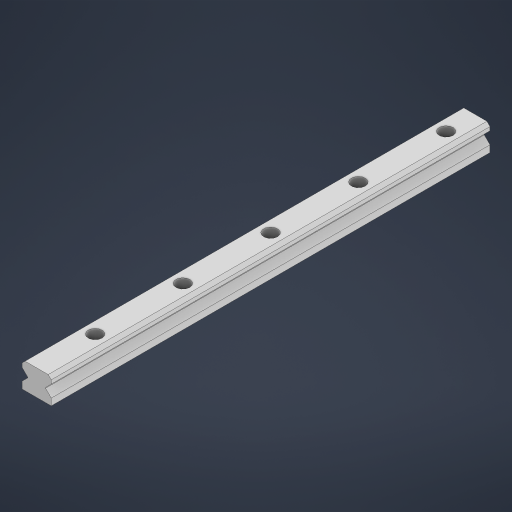
# Autodesk Inventor part: HGR20 500mm
Saved by Autodesk Inventor 2024.2 (Build 282272000, 272)
## iProperties
Created: 2024-10-04
Part Number: HGR20 500mm
Material: Generic
Document SubType Name: Modeling
Designer: jerem
Density: 1 g/cm^3
Appearance: Default
Author: jerem
Autodesk Inventor part; units mm, degrees
ref_plane "YZ Plane" through (0, 0, 0) normal (1, 0, 0) x (0, 1, 0)
ref_plane "XZ Plane" through (0, 0, 0) normal (0, 1, 0) x (-1, 0, 0)
ref_plane "XY Plane" through (0, 0, 0) normal (0, 0, 1) x (1, 0, 0)
sketch "Sketch1" plane through (0, 0, 0) normal (0, 0, 1) x (1, 0, 0)
  line L0 (0, 0) -> (0, 17.5) construction
  line L1 (0, 0) -> (-10, 0)
  line L2 (0, 0) -> (10, 0)
  line L3 (-10, 0) -> (-10, 4.6)
  line L4 (-10, 4.6) -> (-6.1, 8.5)
  line L5 (-6.1, 8.5) -> (-6.1, 9)
  line L6 (-6.1, 9) -> (-10, 12.9)
  line L7 (-10, 12.9) -> (-10, 15.4)
  line L8 (-10, 15.4) -> (-7.9, 17.5)
  line L9 (-7.9, 17.5) -> (0, 17.5)
  line L10 (10, 0) -> (10, 4.6)
  line L11 (10, 4.6) -> (6.1, 8.5)
  line L12 (6.1, 8.5) -> (6.1, 9)
  line L13 (6.1, 9) -> (10, 12.9)
  line L14 (10, 12.9) -> (10, 15.4)
  line L15 (10, 15.4) -> (7.9, 17.5)
  line L16 (7.9, 17.5) -> (0, 17.5)
  dimension "d0" = 17.5
  dimension "d1" = 20
  dimension "d2" = 4.6
  dimension "d3" = 8.5
  dimension "d8" = 135
  dimension "d9" = 0.5
  dimension "d10" = 135
  dimension "d11" = 2.5
  constraints: 34 end point, 6 symmetric about line, 4 point on line, 2 horizontal, 2 parallel, 2 vertical, 1 collinear, 1 perpendicular
  measures "d0" distance of L0.start L0.end
  measures "d1" distance of L2.end L1.end
  measures "d2" distance of L1.end L3.end
  measures "d3" distance from line of L5.end L9
  measures "d8" angle of L9 L8
  measures "d9" distance of L4.end L5.end
  measures "d10" angle of L5 L6
  measures "d11" distance of L6.end L7.end
extrude "Extrusion1" add sketch "Sketch1" along normal blind 300
sketch "Sketch2" plane through (0, 0, 0) normal (0, 1, 0) x (-1, 0, 0)
  line L0 (0, 0) -> (0, 20) construction
  line L1 (0, 20) -> (0, 80) construction
  circle A0 centre (0, 20) radius 4.75
  circle A1 centre (0, 20) radius 3
  dimension "d14" = 20
  dimension "d15" = 60
  dimension "d16" = 9.5
  dimension "d17" = 6
  constraints: 4 end point, 2 centre point, 2 coincident, 1 point on line, 1 vertical
  measures "d14" distance of L0.start L0.end
  measures "d15" distance of L0.end L1.end
  measures "d16" diameter of A0
  measures "d17" diameter of A1
extrude "Extrusion2" cut sketch "Sketch2" along normal through all contours A1
extrude "Extrusion3" cut sketch "Sketch2" against normal blind 8.5 from surface at 17.5
pattern_linear "Rectangular Pattern1" count 9 spacing 60 along (0, 0, 1) of "Extrusion2", "Extrusion3"
body "Solid1"
